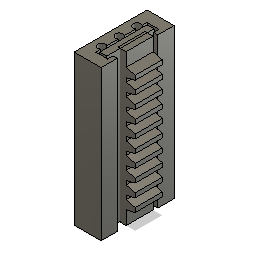
SuspensionRack (Autodesk Fusion 360 design; units mm, degrees)
Autodesk Fusion 360 part; units mm, degrees
sketch "Sketch1" plane through (0, 0, 0) normal (0, 0, 1) x (1, 0, 0)
  spline S0 degree 5 poles (-8.7331, -2.7764) (-8.7326, -2.782) (-8.7316, -2.7932) (-8.7296, -2.8099) (-8.7261, -2.8321) (-8.7208, -2.8598) (-8.7146, -2.8873) (-8.708, -2.9148) (-8.7011, -2.9423) (-8.694, -2.9697) (-8.6868, -2.9972) (-8.6793, -3.0246) (-8.6715, -3.052) (-8.6633, -3.0793) (-8.6547, -3.1065) (-8.6458, -3.1337) (-8.6366, -3.1609) (-8.6272, -3.188) (-8.6175, -3.2151) (-8.6076, -3.2421) (-8.5976, -3.2691) (-8.5873, -3.2961) (-8.5768, -3.3231) (-8.566, -3.35) (-8.555, -3.3768) (-8.5438, -3.4037) (-8.5324, -3.4304) (-8.5208, -3.4572) (-8.509, -3.4839) (-8.497, -3.5106) (-8.4848, -3.5372) (-8.4725, -3.5638) (-8.4599, -3.5903) (-8.4472, -3.6169) (-8.4342, -3.6433) (-8.4211, -3.6698) (-8.4079, -3.6962) (-8.3944, -3.7225) (-8.3808, -3.7489) (-8.367, -3.7751) (-8.353, -3.8014) (-8.3389, -3.8276) (-8.3246, -3.8538) (-8.3101, -3.8799) (-8.2955, -3.906) (-8.2807, -3.932) (-8.2658, -3.958) (-8.2507, -3.984) (-8.2355, -4.0099) (-8.2201, -4.0358) (-8.2045, -4.0617) (-8.1888, -4.0875) (-8.173, -4.1132) (-8.1569, -4.139) (-8.1408, -4.1646) (-8.1245, -4.1903) (-8.1081, -4.2159) (-8.0915, -4.2414) (-8.0747, -4.2669) (-8.0579, -4.2924) (-8.0408, -4.3178) (-8.0237, -4.3432) (-8.0064, -4.3686) (-7.989, -4.3939) (-7.9714, -4.4191) (-7.9537, -4.4443) (-7.9358, -4.4695) (-7.9178, -4.4946) (-7.8997, -4.5197) (-7.8815, -4.5447) (-7.8631, -4.5697) (-7.8483, -4.5897) (-7.8371, -4.6046) (-7.8297, -4.6146) (-7.8259, -4.6195) knots 0 0 0 0 0 0 0.01428571 0.02857143 0.04285714 0.05714286 0.07142857 0.08571429 0.1 0.11428571 0.12857143 0.14285714 0.15714286 0.17142857 0.18571429 0.2 0.21428571 0.22857143 0.24285714 0.25714286 0.27142857 0.28571429 0.3 0.31428571 0.32857143 0.34285714 0.35714286 0.37142857 0.38571429 0.4 0.41428571 0.42857143 0.44285714 0.45714286 0.47142857 0.48571429 0.5 0.51428571 0.52857143 0.54285714 0.55714286 0.57142857 0.58571429 0.6 0.61428571 0.62857143 0.64285714 0.65714286 0.67142857 0.68571429 0.7 0.71428571 0.72857143 0.74285714 0.75714286 0.77142857 0.78571429 0.8 0.81428571 0.82857143 0.84285714 0.85714286 0.87142857 0.88571429 0.9 0.91428571 0.92857143 0.94285714 0.95714286 0.97142857 0.98571429 1 1 1 1 1 1
  line L0 (-8.7786, -2.2245) -> (-8.7331, -2.7764)
  arc A0 (-8.7786, -2.2245) -> (-9.6845, -1.3986) centre (-9.6756, -2.2986) ccw
  circle A1 centre (-9.8, 10.25) radius 13.5 construction
  line L1 (-29.9989, -3.25) -> (11.6191, -3.25) construction
  line L2 (-9.8, -1.4) -> (-9.8, -5.0546) construction
  line L3 (-9.8, -3.25) -> (-7.2731, -2.5965) construction
  line L4 (-9.8, -3.25) -> (-7.1899, -3.25)
  circle A2 centre (-9.8, -3.25) radius 1.141 construction
  circle A3 centre (-9.8, -3.25) radius 1.141 construction
  line L5 (-29.9989, -5.125) -> (11.6191, -5.125) construction
  line L6 (-29.9989, -1.75) -> (11.6191, -1.75) construction
  line L7 (-10.5906, -1.75) -> (-11.4634, -5.125)
  line L8 (-9.0094, -1.75) -> (-8.1366, -5.125)
  line L9 (-10.5906, -1.75) -> (-9.0094, -1.75)
  line L10 (-11.4634, -5.125) -> (-8.1366, -5.125)
  point P0 (-8.6954, -2.9643)
  dimension "d455" = 27
  dimension "d457" = 14.5
  dimension "d458" = 2.6101
  dimension "d460" = 1.875
  dimension "d462" = 14.5
  dimension "d463" = 14.5
  constraint horizontal L1
  constraint tangent A1 L1
  constraint vertical L2
  constraint horizontal L4
  constraint coincident L2 L3.start
  constraint coincident A1 L3.start
  constraint coincident S0 P0
  constraint coincident L3 P0
  constraint coincident L3.start L4.start
  constraint coincident P0 A2
  constraint coincident L6 L7.start
  constraint coincident L5 L7.end
  constraint tangent A3 L7
  constraint coincident L6 L8.start
  constraint coincident L5 L8.end
  constraint tangent A3 L8
  constraint perpendicular L2 L9
  constraint perpendicular L2 L10
  measures "d455" diameter of A1
  measures "d457" angle of L3 L4
  measures "d458" distance of L3.start L3.end
  measures "d462" angle of L2 L7
  measures "d463" angle of L2 L8
extrude "Extrude1" add sketch "Sketch1" against normal blind 10 contours L7 L8 L9 L10 makes body 1
pattern_linear "R-Pattern1" count 10 spacing 4.7124 along (1, 0, 0) of bodies 1 makes body 2 at (-6.1691, -2.875, -3.3333) makes body 3 at (-1.4567, -2.875, -3.3333) makes body 4 at (3.2557, -2.875, -3.3333) makes body 5 at (7.968, -2.875, -3.3333) makes body 6 at (12.6804, -2.875, -3.3333) makes body 7 at (17.3928, -2.875, -3.3333) makes body 8 at (22.1052, -2.875, -3.3333) makes body 9 at (26.8176, -2.875, -3.3333) makes body 10 at (31.53, -2.875, -3.3333)
sketch "Sketch2" plane through (0, 0, 0) normal (0, 0, 1) x (1, 0, 0)
  line L0 (-10.5906, -1.75) -> (-11.4634, -5.125)
  line L1 (-11.4634, -5.125) -> (-8.1366, -5.125)
  line L2 (-8.1366, -5.125) -> (-9.0094, -1.75)
  line L3 (-9.0094, -1.75) -> (-10.5906, -1.75)
  line L4 (-11.4634, -5.125) -> (-16.4634, -5.125)
  line L5 (-8.1366, -5.125) -> (39.2749, -5.125)
  line L6 (39.2749, -5.125) -> (39.2749, -8.125)
  line L7 (39.2749, -8.125) -> (-16.4634, -8.125)
  line L8 (-16.4634, -8.125) -> (-16.4634, -5.125)
  dimension "d470" = 5
  dimension "d471" = 47.4115
  dimension "d472" = 3
  constraint horizontal L4
  constraint coincident L0.end L1.start
  constraint horizontal L5
  constraint coincident L1.end L2.start
  constraint perpendicular L5 L6
  constraint perpendicular L6 L7
  constraint perpendicular L4 L8
  measures "d470" distance of L0.end L4.end
  measures "d471" distance of L1.end L5.end
  measures "d472" distance of L5.end L6.end
extrude "Extrude2" add sketch "Sketch2" against normal blind 10 contours L1 L4 L5 L6 L7 L8 bodies 1 2 3 4 5 6 7 8 9 10
move_body "Move1" bodies 1 to x (0, -1, 0) y (1, 0, 0) z (0, 0, 1) at (-20.1835, 35.8065, 0)
move_body "Move3" bodies 1 to x (1, 0, 0) y (0, 1, 0) z (0, 0, 1) at (0, 0, 5)
ref_plane "WorkPlane1" through (-26.8085, -3.4784, 0) normal (0, -1, 0) x (-1, 0, 0)
sketch "Sketch3" plane through (-27.8085, -3.4784, -5) normal (0, -1, 0) x (1, 0, 0)
  line L0 (3, 14.7) -> (-3, 14.7)
  line L1 (-3, 14.7) -> (-3, -4.3)
  line L2 (-3, -4.3) -> (3, -4.3)
  line L3 (3, -4.3) -> (3, -8.3)
  line L4 (3, -8.3) -> (-7, -8.3)
  line L5 (-7, -8.3) -> (-7, 18.7)
  line L6 (-7, 18.7) -> (3, 18.7)
  line L7 (3, 18.7) -> (3, 14.7)
  line L8 (1.4, -4.3) -> (1.4, -2.3)
  line L9 (1.4, -2.3) -> (3, -2.3)
  line L10 (3, -2.3) -> (3, -4.3)
  line L11 (1.4, 14.7) -> (1.4, 12.7)
  line L12 (1.4, 12.7) -> (3, 12.7)
  line L13 (3, 12.7) -> (3, 14.7)
  circle A0 centre (-3.8, -1.3) radius 1.4
  circle A1 centre (-3.8, 11.7) radius 1.4
  circle A2 centre (-3.8, 5.2) radius 1.4
  dimension "d501" = 10
  dimension "d502" = 27
  dimension "d570" = 1.6
  dimension "d571" = 90
  dimension "d572" = 4.4
  dimension "d573" = 1.6
  dimension "d574" = 90
  dimension "d575" = 4.4
  dimension "d586" = 2
  dimension "d588" = 2
  dimension "d595" = 4
  dimension "d596" = 2.8
  dimension "d597" = 3
  dimension "d598" = 3.2
  dimension "d599" = 2.8
  dimension "d600" = 3.2
  dimension "d601" = 3
  dimension "d602" = 4
  dimension "d603" = 2.8
  dimension "d606" = 6.5
  dimension "d613" = 3.2
  dimension "d614" = 6.4
  constraint horizontal L0
  constraint perpendicular L0 L1
  constraint perpendicular L1 L2
  constraint perpendicular L2 L3
  constraint perpendicular L1 L4
  constraint perpendicular L0 L5
  constraint perpendicular L5 L6
  constraint perpendicular L0 L7
  constraint coincident L2 L8.start
  constraint perpendicular L2 L8
  constraint perpendicular L8 L9
  constraint coincident L2 L3.start
  constraint coincident L0 L11.start
  constraint perpendicular L0 L11
  constraint perpendicular L11 L12
  constraint coincident L0 L7.end
  measures "d501" distance of L3.end L4.end
  measures "d502" distance of L4.end L5.end
  measures "d570" distance of L8.end L9.end
  measures "d571" angle of L9 L10
  measures "d572" distance of L1 L8
  measures "d573" distance of L11.end L12.end
  measures "d574" angle of L12 L13
  measures "d575" distance of L1 L11
  measures "d586" distance of L9.end L2.end
  measures "d588" distance of L12.end L0.start
  measures "d595" distance of L0.start L6.end
  measures "d596" diameter of A0
  measures "d597" distance of L2 A0.centre
  measures "d598" distance of L5 A0.centre
  measures "d599" diameter of A1
  measures "d600" distance of L5 A1.centre
  measures "d601" distance of L0 A1.centre
  measures "d602" distance of L2.end L3.end
  measures "d603" diameter of A2
  measures "d606" distance of A1.centre A2.centre
  measures "d613" distance of L5 A2.centre
extrude "Extrude3" add sketch "Sketch3" against normal blind 55.5 separate body contours L0 L11 L12 L13 | L0 L1 L2 L3 L4 L5 L6 L7 A0 A1 A2 | L2 L8 L9 L10 makes body 11
copy_body "Body->Comp1" bodies 11 removing the originals makes body 12 in component "RackGuide"
copy_body "Body->Comp2" bodies 1 removing the originals makes body 13 in component "RackTeeth"
move_body "Move1'" bodies 12 to x (1, 0, 0) y (0, 1, 0) z (0, 0, 1) at (-2.5, 0, 3) in component "RackGuide"
move_body "Move1''" bodies 13 to x (1, 0, 0) y (0, 1, 0) z (0, 0, 1) at (1, 0, 0) in component "RackTeeth"
sketch "Sketch6" plane through (0.5, -3.4684, 4) normal (0, -1, 0) x (1, 0, 0)
  line L0 (-25.3085, -17.25) -> (-25.3085, -11.25)
  line L1 (-25.3085, -11.25) -> (-26.9085, -11.25)
  line L2 (-26.9085, -11.25) -> (-26.9085, -13.25)
  line L3 (-26.9085, -13.25) -> (-31.3085, -13.25)
  line L4 (-31.3085, -13.25) -> (-31.3085, -11.3989)
  arc A0 (-31.3085, -9.1011) -> (-31.3085, -11.3989) centre (-32.1085, -10.25) ccw
  line L5 (-31.3085, -9.1011) -> (-31.3085, -4.8989)
  arc A1 (-31.3085, -2.6011) -> (-31.3085, -4.8989) centre (-32.1085, -3.75) ccw
  line L6 (-31.3085, -2.6011) -> (-31.3085, 1.6011)
  arc A2 (-31.3085, 3.8989) -> (-31.3085, 1.6011) centre (-32.1085, 2.75) ccw
  line L7 (-31.3085, 3.8989) -> (-31.3085, 5.75)
  line L8 (-31.3085, 5.75) -> (-26.9085, 5.75)
  line L9 (-26.9085, 5.75) -> (-26.9085, 3.75)
  line L10 (-26.9085, 3.75) -> (-25.3085, 3.75)
  line L11 (-25.3085, 3.75) -> (-25.3085, 9.75)
  line L12 (-25.3085, 9.75) -> (-35.3085, 9.75)
  line L13 (-35.3085, 9.75) -> (-35.3085, -17.25)
  line L14 (-35.3085, -17.25) -> (-25.3085, -17.25)
  line L15 (-27.9585, 5) -> (-30.5585, 5)
  line L16 (-30.5585, 5) -> (-30.5585, -12.5)
  line L17 (-30.5585, -12.5) -> (-27.9585, -12.5)
  line L18 (-27.9585, -12.5) -> (-27.9585, 5)
  dimension "d607" = 2.6
  dimension "d608" = 0.75
  dimension "d609" = 0.75
  dimension "d610" = 0.75
  constraint horizontal L15
  constraint vertical L16
  constraint horizontal L17
  constraint vertical L18
  measures "d607" distance of L15.start L15.end
  measures "d608" distance of L7 L16
  measures "d609" distance of L8 L15
  measures "d610" distance of L3 L17
extrude "Extrude5" add sketch "Sketch6" against normal blind 55.5 separate body contours L15 L16 L17 L18 makes body 14
copy_body "Body->Comp3" bodies 14 removing the originals makes body 15 in component "RackTeethBase"
component "RackGuide" placed x (1, 0, 0) y (0, -1, 0) z (0, 0, -1) at (2.5, 48.5533, 3.45)
component "RackTeeth" placed x (1, 0, 0) y (0, -1, 0) z (0, 0, -1) at (-1, 48.5533, -1)
component "RackTeethBase" placed x (1, 0, 0) y (0, 1, 0) z (0, 0, 1) at (0, 0, 0)
equation "d455 = pitchcirclediam"
equation "d457 = pressureangle"
equation "d459 = -backlash"
equation "d460 = dedendum"
equation "d461 = -addendum"
equation "d462 = pressureangle"
equation "d463 = pressureangle"
equation "d464 = -thickness"
equation "d466 = rackteeth"
equation "d468 = racktoothpitch"
equation "d471 = spurteeth * racktoothpitch / 2 + 5 mm"
equation "d473 = -thickness"
equation "diametralpitch = 6.666666666666667 cm"
equation "spurteeth = 18"
equation "pressureangle = 14.5 deg"
equation "thickness = 1 cm"
equation "pitchcirclediam = ( spurteeth / diametralpitch * 1 cm ) * 1 cm"
equation "backlash = 0 cm"
equation "addendum = ( 1 / diametralpitch * 1 cm ) * 1 cm"
equation "dedendum = ( 1.25 / diametralpitch * 1 cm ) * 1 cm"
equation "rackteeth = 10"
equation "racktoothpitch = ( PI / diametralpitch * 1 cm ) * 1 cm"
named bodies: "RackTeeth", "RackGuideRail", "RackTeeth (1)", "RackTeethBase"
